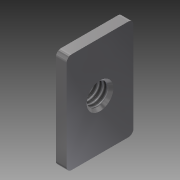
# Autodesk Inventor part: HNKK5-4
Saved by Autodesk Inventor 2016 (Build 200138000, 138)
## iProperties
Category: Hardware
Company: MISUMI
Created: 2015-03-14
Part Number: HNKK5-4
Catalog Web Link: http://us.misumi-ec.com/vona2/detail/110302246940/
Description: HNKK-Pre-Assembly Square Nuts for Aluminum Frames
Vendor: MISUMI
Document SubType Name: Modeling
Designer: PARTuser1
Manufacturer: MISUMI
Mass: 2.05027 g
Surface Area: 4.17218 cm^2
Volume: 0.265235 cm^3
Density: 7.73 g/cm^3
Material: Steel, Alloy
Appearance: Semi-Polished
Stock Number: HNKK5-4
PSOL_IDENT_0: {\\10.0.0.236\data_v8\23d-libs\misumi\metric\38_al_extrusions_blackets\nuts\hnkk.prj},155 {VTYP=3D},
PSOL_IDENT_1: {NB=HNKK5-4},{LINA=HNKK5-4},{NN=HNKK},{DATE=02.02.2015 06:12:46},{GEOMDATE=05.03.2008 07:18:00},{VER
PSOL_IDENT_2: SION=},{LINEID=10},{LINESUBID=-1},{WBVAR=M}  {NB=HNKK5-4},{LINA=HNKK5-4},{KT=DUMMY},{PN=HNKK5-4},{TP=
PSOL_IDENT_3: HNKK},{MAT=SPCC (Low Carbon Steel)(1.0330_DC01(St.12)or 1.0320_St.22)},{ST=Trivalent Chromate},{NO=5
PSOL_IDENT_4: },{M=4},{MA= '3' , '4' , '5' },{MN=4},{CFSW=6},{AFS=HFS5},{B=10.0},{L=15.0},{E=1.6},{T=3.0},{D=6.9}
SUPPLIER: MISUMI
ARTICLENO: HNKK5-4
BOMINFO: HNKK5-4
CREATOR: CADENAS GmbH
Title: HNKK5-4
Author: Misumi
Autodesk Inventor part; units mm, degrees
ref_plane "YZ Plane" through (0, 0, 0) normal (1, 0, 0) x (0, 1, 0)
ref_plane "XZ Plane" through (0, 0, 0) normal (0, 1, 0) x (-1, 0, 0)
ref_plane "XY Plane" through (0, 0, 0) normal (0, 0, 1) x (1, 0, 0)
sketch "Sketch_1" plane through (0, 0, 0) normal (1, 0, 0) x (0, 1, 0)
  line L0 (4.25, 7.5) -> (-4.25, 7.5)
  arc A0 (-4.25, 7.5) -> (-5, 6.75) centre (-4.25, 6.75) ccw
  line L1 (-5, 6.75) -> (-5, -6.75)
  arc A1 (-5, -6.75) -> (-4.25, -7.5) centre (-4.25, -6.75) ccw
  line L2 (-4.25, -7.5) -> (4.25, -7.5)
  arc A2 (4.25, -7.5) -> (5, -6.75) centre (4.25, -6.75) ccw
  line L3 (5, -6.75) -> (5, 6.75)
  arc A3 (5, 6.75) -> (4.25, 7.5) centre (4.25, 6.75) ccw
  constraints: 8 end point, 8 point on circle, 4 centre point
extrude "Extrusion1" add sketch "Sketch_1" against normal blind 3
sketch "Sketch_2" plane through (0, 0, 0) normal (0, 0, 1) x (1, 0, 0)
  line L0 (3, 0) -> (-3, 0)
  line L1 (-4.6, 3.45) -> (-1.6, 3.45)
  line L2 (-1.6, 3.45) -> (-1.6, 13.45)
  line L3 (-1.6, 13.45) -> (-4.6, 13.45)
  line L4 (-4.6, 13.45) -> (-4.6, 3.45)
  constraints: 10 end point
revolve "Revolution1" cut sketch "Sketch_2" angle 360 about axis through (3, 0, 0) along (1, 0, 0)
sketch "Sketch_3" plane through (0, 0, 0) normal (0, 0, 1) x (1, 0, 0)
  line L0 (0, 0) -> (-3, 0)
  line L1 (-3, 0) -> (-3, 2)
  line L2 (-3, 2) -> (-2.621, 1.621)
  line L3 (-2.621, 1.621) -> (-0.379, 1.621)
  line L4 (-0.379, 1.621) -> (0, 2)
  line L5 (0, 2) -> (0, 0)
  line L6 (0, 0) -> (-3, 0)
  constraints: 14 end point
revolve "Revolution2" cut sketch "Sketch_3" angle 360 about axis through (0, 0, 0) along (1, 0, 0)
thread "Thread1" size "M4x0.7" class "6H" standard "ISO Metric profile" full length
ref_plane "dummy_XY" through (0, 0, 0) normal (1, 0, 0) x (0, 0, -1)
ref_plane "dummy_YZ" through (0, 0, 0) normal (0, 0, -1) x (0, 1, 0)
ref_plane "dummy_ZX" through (0, 0, 0) normal (0, 1, 0) x (1, 0, 0)
body "Solid1"
